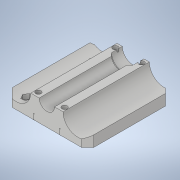
# Autodesk Inventor part: MINI-z-carriage-rear
Saved by Autodesk Inventor 2021 (Build 250183000, 183)
## iProperties
Company: Prusa Development a.s.
RuleStatus: InUse
Created: 2019-07-11
Material: Všeobecné
Document SubType Name: Modeling
Density: 1 g/cm^3
Appearance: Výchozí
Project: ORIGINAL PRUSA MINI
Authority: Ing. Robert Turinský
Author: Ing. Robert Turinský
Title: MINI-z-carriage-rear
Revision Number: R4
Autodesk Inventor part; units mm, degrees
ref_plane "YZ Plane" through (0, 0, 0) normal (1, 0, 0) x (0, 1, 0)
ref_plane "XZ Plane" through (0, 0, 0) normal (0, 1, 0) x (-1, 0, 0)
sketch "Náčrt1" plane through (0, 0, 0) normal (0, 0, 1) x (1, 0, 0)
  line L0 (0, -16.8) -> (0, 2.8) projected
  line L1 (-37.1, 0) -> (37.1, 0) projected
  arc A0 (-5, 0) -> (5, 0) centre (0, 0) ccw
  arc A1 (-26.5, -6.9282) -> (-10.5, 0) centre (-20, 0) ccw
  arc A2 (10.5, 0) -> (26.5, -6.9282) centre (20, 0) ccw
  line L2 (-10.5, 0) -> (-5, 0)
  line L3 (5, 0) -> (10.5, 0)
  line L4 (-26.5, -6.9282) -> (-26.5, -14)
  line L5 (-26.5, -14) -> (26.5, -14)
  line L6 (26.5, -14) -> (26.5, -6.9282)
  dimension "d0" = 19
  dimension "d1" = 10
  dimension "d2" = 40
  dimension "d3" = 53
  dimension "d4" = 14
  constraints: 10 end point, 6 point on circle, 3 centre point, 2 vertical, 1 coincident, 1 equal radius, 1 horizontal, 1 symmetric about line, 8 other
  measures "d0" diameter of A1
  measures "d1" diameter of A0
  measures "d2" distance of A2.centre A1.centre
  measures "d3" distance between parallel lines of L6 L4
  measures "d4" distance of the line from the sketch origin of L5
extrude "Vysunutí1" add sketch "Náčrt1" along normal mid plane 56 contours L5 L4 A1 L1 A0 L0 | L0 A0 L1 A2 L6 L5
sketch "Náčrt2" plane through (0, 0, -28) normal (0, 0, -1) x (-1, 0, 0)
  circle A0 centre (0, 0) radius 7
  point P0 (0, -9.5)
  dimension "d7" = 14
  dimension "d13" = 9.5
  constraints: 1 centre point, 1 coincident, 1 vertical alignment
  measures "d7" diameter of A0
  measures "d13" distance of point (0, 0) point (0, -9.5)
extrude "Vysunutí2" cut sketch "Náčrt2" against normal blind 7
chamfer "Zkosení1" distance 2 angle 45 1 edges at (0, -5, -21)
hole "Díra1" at (0, -9.5, -28) direction (0, 0, 1) diameter 3.4 depth 16 countersink diameter 4 countersink angle 60
sketch "Náčrt4" plane through (-26.5, -14, 28) normal (0, -1, 0) x (1, 0, 0)
  line L0 (26.5, -67.2) -> (26.5, 11.2) projected
  line L1 (-10.6, -28) -> (63.6, -28) projected
  line L2 (53, -56) -> (0, -56) projected
  line L3 (0, 0) -> (53, 0) projected
  point P0 (26.5, -28)
  point P1 (18, -3)
  point P2 (35, -3)
  point P3 (18, -53)
  point P4 (35, -53)
  dimension "d24" = 17
  dimension "d25" = 3
  dimension "d121" = 50
  constraints: 2 symmetric about line, 1 vertical alignment
  measures "d24" distance of point (35, -53) point (18, -53)
  measures "d25" distance from line of point (35, -53) L2
  measures "d121" distance of point (35, -3) point (35, -53)
hole "Díra2" at (-8.5, -14, 25) at (8.5, -14, 25) at (-8.5, -14, -25) at (8.5, -14, -25) direction (0, 1, 0) diameter 3.4 end through all counterbore diameter 6 counterbore depth 4.1
ref_plane "Pracovní rovina1" through (-26.5, -12.5, 28) normal (0, -1, 0) x (1, 0, 0)
sketch "Náčrt5" plane through (-26.5, -12.5, 28) normal (0, -1, 0) x (1, 0, 0)
  line L0 (26.5, -67.2) -> (26.5, 11.2) projected
  line L1 (-10.6, -28) -> (63.6, -28) projected
  circle A0 centre (8, -6) radius 1.7
  line L2 (0, 0) -> (53, 0) projected
  circle A1 centre (9.5, -48) radius 1.7
  line L3 (9.6166, -3.2) -> (11.2332, -6)
  line L4 (11.2332, -6) -> (9.6166, -8.8)
  line L5 (9.6166, -8.8) -> (6.3834, -8.8)
  line L6 (6.3834, -8.8) -> (4.7668, -6)
  line L7 (4.7668, -6) -> (6.3834, -3.2)
  line L8 (6.3834, -3.2) -> (9.6166, -3.2)
  line L9 (11.1166, -45.2) -> (12.7332, -48)
  line L10 (12.7332, -48) -> (11.1166, -50.8)
  line L11 (11.1166, -50.8) -> (7.8834, -50.8)
  line L12 (7.8834, -50.8) -> (6.2668, -48)
  line L13 (6.2668, -48) -> (7.8834, -45.2)
  line L14 (7.8834, -45.2) -> (11.1166, -45.2)
  point P0 (26.5, -28)
  dimension "d35" = 3.4
  dimension "d36" = 18.5
  dimension "d37" = 6
  dimension "d38" = 42
  dimension "d39" = 17
  dimension "d40" = 5.6
  constraints: 24 end point, 2 centre point, 2 coincident, 2 horizontal, 1 equal radius, 1 parallel, 26 other
  measures "d35" diameter of A0
  measures "d36" distance from line of L0 A0.centre
  measures "d37" distance from line of L2 A0.centre
  measures "d38" vertical distance of A1.centre A0.centre
  measures "d39" distance from line of L0 A1.centre
  measures "d40" distance between parallel lines of L5 L8
extrude "Vysunutí3" cut sketch "Náčrt5" along normal through all contours A0 | A1
extrude "Vysunutí4" cut sketch "Náčrt5" against normal through all contours A0 | A1 | L3 L4 L5 L6 L7 L8 | L9 L10 L11 L12 L13 L14
sketch "Náčrt6" plane through (-26.5, -14, 28) normal (0, -1, 0) x (1, 0, 0)
  circle A0 centre (47.5, -11) radius 3.25
  circle A1 centre (41.9, -44.9) radius 1.5
  circle A2 centre (4.5, -12) radius 1.5
  line L0 (26.5, -67.2) -> (26.5, 11.2) projected
  line L1 (-10.6, -28) -> (63.6, -28) projected
  line L2 (0, 0) -> (53, 0) projected
  point P0 (26.5, -28)
  dimension "d45" = 6.5
  dimension "d46" = 22
  dimension "d47" = 12
  dimension "d48" = 3
  dimension "d49" = 21
  dimension "d50" = 11
  dimension "d51" = 15.4
  dimension "d52" = 44.9
  dimension "d53" = 3
  constraints: 3 centre point
  measures "d45" diameter of A0
  measures "d46" distance from line of L0 A2.centre
  measures "d47" distance from line of A2.centre L2
  measures "d48" diameter of A2
  measures "d49" distance from line of L0 A0.centre
  measures "d50" distance from line of L2 A0.centre
  measures "d51" distance from line of L0 A1.centre
  measures "d52" distance from line of L2 A1.centre
  measures "d53" diameter of A1
extrude "Vysunutí5" cut sketch "Náčrt6" against normal blind 2 contours A1 | A2
extrude "Vysunutí6" cut sketch "Náčrt6" against normal blind 3 contours A0
chamfer "Zkosení2" distance 4 angle 45 2 edges at (-26.5, -10.4641, 28) (26.5, -10.4641, 28)
chamfer "Zkosení3" distance 5.5 angle 45 1 edges at (26.5, -10.4641, -28)
chamfer "Zkosení4" distance 1.5 angle 45 1 edges at (-26.5, -10.4641, -28)
ref_plane "Pracovní rovina2" through (0, 0, -18) normal (0, 0, -1) x (-1, 0, 0)
sketch "Náčrt7" plane through (0, 0, -18) normal (0, 0, -1) x (-1, 0, 0)
  line L0 (-17.75, -14) -> (-24.25, -14) projected
  line L1 (-13.9, -14) -> (-16.9, -14) projected
  line L2 (23.5, -14) -> (20.5, -14) projected
  line L3 (20.2, -14) -> (16.8, -14) projected
  line L4 (18.7, -14) -> (15.3, -14) projected
  line L5 (11.5, -14) -> (5.5, -14) projected
  line L6 (11.5, -14) -> (5.5, -14) projected
  line L7 (-5.5, -14) -> (-11.5, -14) projected
  line L8 (-5.5, -14) -> (-11.5, -14) projected
  line L9 (25, -14) -> (26.5, -14) projected
  line L10 (-21, -14) -> (-8.5, -14) projected
  line L11 (-26.5, -14) -> (-21, -14) projected
  line L12 (-22.5, -14) -> (-26.5, -14) projected
  line L13 (22.5, -14) -> (8.5, -14) projected
  line L14 (26.5, -14) -> (22.5, -14) projected
  circle A0 centre (0, -9.5) radius 1.7 projected
  line L15 (22.5, -14) -> (-22.5, -14) projected
  line L16 (2.8, -14) -> (-2.8, -14)
  line L17 (-2.8, -14) -> (-2.8, -6.7)
  line L18 (-2.8, -6.7) -> (2.8, -6.7)
  line L19 (2.8, -6.7) -> (2.8, -14)
  line L20 (2.8, -14) -> (1.7, -14)
  line L21 (1.7, -14) -> (1.7, -6.7)
  line L22 (1.7, -6.7) -> (2.8, -6.7)
  line L23 (2.8, -6.7) -> (2.8, -14)
  line L24 (2.8, -6.7) -> (-2.8, -6.7)
  line L25 (-2.8, -6.7) -> (-2.8, -7.8)
  line L26 (-2.8, -7.8) -> (2.8, -7.8)
  line L27 (2.8, -7.8) -> (2.8, -6.7)
  line L28 (-2.8, -6.7) -> (-1.7, -6.7)
  line L29 (-1.7, -6.7) -> (-1.7, -14)
  line L30 (-1.7, -14) -> (-2.8, -14)
  line L31 (-2.8, -14) -> (-2.8, -6.7)
  line L32 (-2.8, -14) -> (2.8, -14)
  line L33 (2.8, -14) -> (2.8, -11.2)
  line L34 (2.8, -11.2) -> (-2.8, -11.2)
  line L35 (-2.8, -11.2) -> (-2.8, -14)
  line L36 (-8.5, -14) -> (-22.5, -14) projected
  line L37 (8.5, -14) -> (-8.5, -14) projected
  line L38 (8.5, -14) -> (25, -14) projected
  line L39 (-8.5, -14) -> (8.5, -14) projected
  point P0 (0, 0)
  point P1 (0, -14)
  dimension "d68" = 5.6
  dimension "d69" = 2.8
  constraints: 40 end point, 10 parallel, 5 horizontal, 5 perpendicular, 4 point on line, 4 tangent, 1 midpoint, 1 vertical alignment, 2 other
  measures "d68" distance of L17.end L18.end
  measures "d69" distance from line of L18 A0.centre
extrude "Vysunutí7" cut sketch "Náčrt7" along normal blind 2.6
extrude "Vysunutí8" add sketch "Náčrt7" along normal blind 0.3 contours L21 L26 L19 L34 | L34 L19 L15 L21 | L21 L18 L19 L26 | L29 L34 L17 L26 | L26 L17 L18 L29 | L29 L15 L17 L34
extrude "Vysunutí9" add sketch "Náčrt7" along normal blind 0.6 contours L26 L29 L18 L21 | L34 L21 L15 L29 | L34 L19 L15 L21 | L21 L18 L19 L26 | L26 L17 L18 L29 | L29 L15 L17 L34
chamfer "Zkosení5" distance 0.5 angle 60 4 edges at (2.8, -14, -19.6) (0, -14, -20.6) (-2.8, -14, -19.6) (0, -14, -18.6) measured on face at (0, -14, -18.5) measured on face at (0, -14, -21.1) measured on face at (-3.3, -14, -19.6) measured on face at (3.3, -14, -19.6)
ref_plane "Pracovní rovina3" through (0, 0, 16) normal (0, 0, 1) x (1, 0, 0)
sketch "Náčrt8" plane through (0, 0, 16) normal (0, 0, 1) x (1, 0, 0)
  line L0 (24.25, -14) -> (17.75, -14) projected
  line L1 (16.9, -14) -> (13.9, -14) projected
  line L2 (-20.5, -14) -> (-23.5, -14) projected
  line L3 (-16.8, -14) -> (-20.2, -14) projected
  line L4 (-15.3, -14) -> (-18.7, -14) projected
  line L5 (-5.5, -14) -> (-11.5, -14) projected
  line L6 (-5.5, -14) -> (-11.5, -14) projected
  line L7 (11.5, -14) -> (5.5, -14) projected
  line L8 (11.5, -14) -> (5.5, -14) projected
  line L9 (-25, -14) -> (-26.5, -14) projected
  line L10 (21, -14) -> (8.5, -14) projected
  line L11 (26.5, -14) -> (21, -14) projected
  line L12 (22.5, -14) -> (26.5, -14) projected
  line L13 (-22.5, -14) -> (-8.5, -14) projected
  line L14 (-26.5, -14) -> (-22.5, -14) projected
  line L15 (-3.3, -14) -> (3.3, -14) projected
  line L16 (3.3, -14) -> (-3.3, -14) projected
  line L17 (0, -16.8003) -> (0, 2.8017) projected
  line L18 (-37.1, 0) -> (37.1, 0) projected
  line L19 (-2, -12) -> (-2, -14)
  line L20 (-2, -14) -> (-9.75, -14)
  line L21 (21, -14) -> (-25, -14) projected
  line L22 (-9.75, -14) -> (-8.5953, -12)
  line L23 (-8.5953, -12) -> (-2, -12)
  line L24 (8.5, -14) -> (22.5, -14) projected
  line L25 (-8.5, -14) -> (8.5, -14) projected
  line L26 (-8.5, -14) -> (-25, -14) projected
  line L27 (8.5, -14) -> (-8.5, -14) projected
  line L28 (-9.75, -14) -> (-10.9047, -14)
  line L29 (-10.9047, -14) -> (-9.1726, -11)
  line L30 (-9.1726, -11) -> (-2, -11)
  line L31 (-2, -11) -> (-2, -12)
  point P0 (0, 0)
  dimension "d80" = 2
  dimension "d85" = 2
  dimension "d127" = 15.5
  dimension "d128" = 60
  dimension "d139" = 1
  dimension "d140" = 1
  constraints: 16 end point, 3 point on line, 2 parallel, 2 perpendicular, 1 horizontal, 1 other
  measures "d80" distance between parallel lines of L17 L19
  measures "d85" distance between parallel lines of L13 L23
  measures "d127" diameter of L20.end L19
  measures "d128" angle of L5 L22
  measures "d139" distance between parallel lines of L30 L23
  measures "d140" distance between parallel lines of L29 L22
revolve "Rotace1" cut sketch "Náčrt8" angle 360 about axis through (-2, -12, 16) along (0, -1, 0) contours L5 L22 L23 L19 L15 L20
sketch "Náčrt9" plane through (-22.5, -14, 28) normal (0, -1, 0) x (1, 0, 0)
  line L0 (22.5, -67.2) -> (22.5, 11.2) projected
  line L1 (-14.6, -28) -> (59.6, -28) projected
  line L2 (10.878, -17.017) -> (34.122, -17.017) construction
  line L3 (34.122, -17.017) -> (34.122, -38.983) construction
  line L4 (34.122, -38.983) -> (10.878, -38.983) construction
  line L5 (10.878, -38.983) -> (10.878, -17.017) construction
  point P0 (22.5, -28)
  constraints: 4 other
feature "Reliéf1" [suppressed]
chamfer "Zkosení6" [suppressed]
chamfer "Zkosení7" [suppressed]
feature "Reliéf2" [suppressed]
sketch "Náčrt11" plane through (8.5, -9.9, -25) normal (0, -1, 0) x (1, 0, 0)
  circle A0 centre (0, 0) radius 3 projected
  circle A1 centre (0, 0) radius 1.7 projected
  circle A2 centre (-17, 0) radius 3 projected
  circle A3 centre (-17, 0) radius 1.7 projected
  circle A4 centre (-17, 50) radius 3 projected
  circle A5 centre (-17, 50) radius 1.7 projected
  circle A6 centre (0, 50) radius 3 projected
  circle A7 centre (0, 50) radius 1.7 projected
  line L0 (1.7, -2.4718) -> (1.7, 2.4718)
  line L1 (-1.7, 2.4718) -> (-1.7, -2.4718)
  line L2 (-2.4718, -1.7) -> (2.4718, -1.7)
  line L3 (2.4718, 1.7) -> (-2.4718, 1.7)
  arc A8 (1.7, -2.4718) -> (1.7, 2.4718) centre (0, 0) ccw
  arc A9 (2.4718, 1.7) -> (-2.4718, 1.7) centre (0, 0) ccw
  arc A10 (-1.7, 2.4718) -> (-1.7, -2.4718) centre (0, 0) ccw
  arc A11 (-2.4718, -1.7) -> (2.4718, -1.7) centre (0, 0) ccw
  point P0 (-8.5, 25)
  point P1 (0, 53)
  point P2 (-17, 53)
  point P3 (-17, -3)
  point P4 (0, -3)
  constraints: 12 point on circle, 8 end point, 4 centre point, 4 tangent, 3 vertical alignment, 2 perpendicular, 2 vertical, 9 other
extrude "Vysunutí10" add sketch "Náčrt11" along normal blind 0.3 contours A0 L2 L0 L3 | L3 L0 A0 | A0 L0 L2 | L1 L3 A0 | A0 L2 L1 | L3 L1 L2 A0
extrude "Vysunutí11" add sketch "Náčrt11" along normal blind 0.6 contours L3 L0 A0 | A0 L0 L2 | L0 L3 L1 A0 | A0 L1 L2 L0 | L1 L3 A0 | A0 L2 L1
pattern_linear "Obdélníkové pole1" count 2 spacing 17 along (-1, 0, 0) count 2 spacing 50 along (0, 0, 1) of "Vysunutí11", "Vysunutí10"
sketch "Náčrt10" plane through (0, 0, -28) normal (0, 0, -1) x (-1, 0, 0)
  line L0 (25, -8.0777) -> (25, -14) projected
  arc A0 (10.5, 0) -> (25, -8.0777) centre (20, 0) ccw projected
  circle A1 centre (0, -9.5) radius 2 projected
  arc A2 (-21, -9.4472) -> (-10.5, 0) centre (-20, 0) ccw projected
  line L1 (-21, -14) -> (-21, -9.4472) projected
  line L2 (-10.5, -7.25) -> (-5.5, -7.25) construction
  line L3 (-5.5, -7.25) -> (-5.5, -12.25) construction
  line L4 (-5.5, -12.25) -> (-10.5, -12.25) construction
  line L5 (-10.5, -12.25) -> (-10.5, -7.25) construction
  line L6 (10.5, 0) -> (7, 0) projected
  arc A3 (-7, 0) -> (7, 0) centre (0, 0) ccw projected
  line L7 (-7, 0) -> (-10.5, 0) projected
  line L8 (-21, -14) -> (-8.5, -14) projected
  line L9 (-8.5, -9.9) -> (-8.5, -14) projected
  line L10 (-8.5, -14) -> (8.5, -14) projected
  line L11 (8.5, -9.9) -> (8.5, -14) projected
  line L12 (8.5, -14) -> (25, -14) projected
  dimension "d95" = 5
  dimension "d97" = 5.5
  constraints: 1 perpendicular, 2 other
  measures "d95" distance of L3.end L4.end
  measures "d97" distance from line of point (0, 0) L3
move faces "Posunout2" translate (0, -2, 0) faces at (-21.8227, -12, 15.5325) (15.8427, -12, -17.1324)
move faces "Posunout3" translate (-1, 0, 0) faces at (24.2395, -13, 17.2615) (19.4208, -11, 16.2816)
sketch "Náčrt12" plane through (-8.5, -14, -28) normal (0, -1, 0) x (1, 0, 0)
  line L0 (8.5, -11.2) -> (8.5, 67.2) projected
  line L1 (-28.6, 28) -> (45.6, 28) projected
  line L2 (-1.9595, 37.5892) -> (18.9595, 37.5892) construction
  line L3 (18.9595, 37.5892) -> (18.9595, 18.4108) construction
  line L4 (18.9595, 18.4108) -> (-1.9595, 18.4108) construction
  line L5 (-1.9595, 18.4108) -> (-1.9595, 37.5892) construction
  line L6 (9.0412, 25.0123) -> (7.2112, 25.0123)
  line L7 (7.2112, 25.0123) -> (5.5463, 27.2112)
  line L8 (5.5463, 27.2112) -> (5.0026, 27.2112)
  line L9 (5.0026, 27.2112) -> (5.0026, 25.0123)
  line L10 (5.0026, 25.0123) -> (3.5075, 25.0123)
  line L11 (3.5075, 25.0123) -> (3.5075, 31.0023)
  line L12 (3.5075, 31.0023) -> (5.9152, 31.0023)
  spline S0 degree 2 poles (5.9152, 31.0023) (6.4152, 31.0023) (7.153, 30.8761) (7.4685, 30.6819) knots 0 0 0 1 2 2 2
  spline S1 degree 2 poles (7.4685, 30.6819) (7.7889, 30.478) (8.1675, 29.8421) (8.1675, 29.3567) knots 0 0 0 1 2 2 2
  spline S2 degree 2 poles (8.1675, 29.3567) (8.1675, 28.6723) (7.5462, 27.8131) (7.0268, 27.5607) knots 0 0 0 1 2 2 2
  line L13 (7.0268, 27.5607) -> (9.0412, 25.0123)
  spline S3 degree 2 poles (6.6239, 29.1674) (6.6239, 29.3956) (6.4491, 29.7208) (6.2501, 29.8082) knots 0 0 0 1 2 2 2
  spline S4 degree 2 poles (6.2501, 29.8082) (6.1093, 29.8664) (5.7647, 29.9004) (5.5074, 29.9004) knots 0 0 0 1 2 2 2
  line L14 (5.5074, 29.9004) -> (5.0026, 29.9004)
  line L15 (5.0026, 29.9004) -> (5.0026, 28.2888)
  line L16 (5.0026, 28.2888) -> (5.4346, 28.2888)
  spline S5 degree 2 poles (5.4346, 28.2888) (5.7453, 28.2888) (6.187, 28.3665) (6.3375, 28.4878) knots 0 0 0 1 2 2 2
  spline S6 degree 2 poles (6.3375, 28.4878) (6.4831, 28.6043) (6.6239, 28.915) (6.6239, 29.1674) knots 0 0 0 1 2 2 2
  line L17 (13.9488, 26.4103) -> (13.1381, 26.4103)
  line L18 (13.1381, 26.4103) -> (13.1381, 24.9977)
  line L19 (13.1381, 24.9977) -> (11.6867, 24.9977)
  line L20 (11.6867, 24.9977) -> (11.6867, 26.4103)
  line L21 (11.6867, 26.4103) -> (9.0461, 26.4103)
  line L22 (9.0461, 26.4103) -> (9.0461, 27.5267)
  line L23 (9.0461, 27.5267) -> (11.6382, 31.0023)
  line L24 (11.6382, 31.0023) -> (13.1381, 31.0023)
  line L25 (13.1381, 31.0023) -> (13.1381, 27.4879)
  line L26 (13.1381, 27.4879) -> (13.9488, 27.4879)
  line L27 (13.9488, 27.4879) -> (13.9488, 26.4103)
  line L28 (11.6867, 27.4879) -> (11.6867, 29.5266)
  line L29 (11.6867, 29.5266) -> (10.1674, 27.4879)
  line L30 (10.1674, 27.4879) -> (11.6867, 27.4879)
  point P0 (8.5, 28)
  dimension "rev_num" = 4
  constraints: 4 other
emboss "Reliéf3" sketch "Náčrt12" operation cut depth 0.75 direction (0, 1, 0) contours L6 L7 L8 L9 L10 L11 L1 S2 L13 L0 | L0 L13 L6 | L1 L11 L12 S0 S1 S2 | L23 L24 L25 L1 L28 L29 | L1 L29 L30 L28 L25 L26 L27 L17 L18 L19 L20 L21 L22 L23
move faces "Posunout4" translate (0, 0, 6.1) faces at (0, -12.4893, -20.6) (-0.9333, -13.7113, -20.9333) (3.1333, -13.7113, -19.9333) (2.8, -10.3447, -19.9333) (-0.9333, -13.7113, -18.2667) (-3.1333, -13.7113, -19.9333) (-0.9333, -6.7, -19.9333) (-2.8, -10.3447, -19.9333) (-0.9333, -7.4333, -18.6) (-0.5667, -7.8, -18.5) (-2.0667, -8.9333, -18.3) (0.9333, -12.4893, -18.6) (-1.7, -9.5, -18.2) (0.5667, -11.2, -18.5) (2.0667, -10.0667, -18.3) (1.7, -9.5, -18.2) (1.363, -10.863, -18) (1.363, -8.137, -18) (-1.363, -8.137, -18) (-1.363, -10.863, -18)
chamfer "Zkosení8" distance 1 angle 45 1 edges at (16.75, -11, 17)
ref_plane "Pracovní rovina4" through (0, 0, -10) normal (0, 0, 1) x (1, 0, 0)
sketch "Náčrt13" plane through (0, 0, -10) normal (0, 0, 1) x (1, 0, 0)
  line L0 (22.5, -9.1652) -> (22.5, -14) projected
  arc A0 (10.5, 0) -> (22.5, -9.1652) centre (20, 0) ccw projected
  line L1 (10.5, 0) -> (5, 0) projected
  arc A1 (-5, 0) -> (5, 0) centre (0, 0) ccw projected
  line L2 (-5, 0) -> (-10.5, 0) projected
  arc A2 (-22.5, -9.1652) -> (-10.5, 0) centre (-20, 0) ccw projected
  line L3 (-22.5, -14) -> (-22.5, -9.1652) projected
  line L4 (-22.5, -14) -> (-8.5, -14) projected
  line L5 (-8.5, -10.5) -> (-8.5, -14) projected
  line L6 (-8.5, -14) -> (8.5, -14) projected
  line L7 (8.5, -10.5) -> (8.5, -14) projected
  line L8 (8.5, -14) -> (22.5, -14) projected
  arc A3 (22.5, -9.1652) -> (26.5, -6.9282) centre (20, 0) ccw projected
  line L9 (22.5, -9.1652) -> (22.5, -14) projected
  line L10 (22.5, -14) -> (26.5, -14) projected
  line L11 (26.5, -14) -> (26.5, -6.9282) projected
  line L12 (-26.5, -14) -> (-22.5, -14) projected
  line L13 (-22.5, -14) -> (-22.5, -9.1652) projected
  arc A4 (-26.5, -6.9282) -> (-22.5, -9.1652) centre (-20, 0) ccw projected
  line L14 (-26.5, -6.9282) -> (-26.5, -14) projected
  line L15 (8.5, -13) -> (21.5, -13)
  line L16 (21.5, -13) -> (21.5, -10.3923)
  arc A5 (9.5477, -1) -> (21.5, -10.3923) centre (20, 0) ccw
  line L17 (9.5477, -1) -> (5.9161, -1)
  arc A6 (-5.9161, -1) -> (5.9161, -1) centre (0, 0) ccw
  line L18 (-5.9161, -1) -> (-9.5477, -1)
  arc A7 (-21.5, -10.3923) -> (-9.5477, -1) centre (-20, 0) ccw
  line L19 (-21.5, -10.3923) -> (-21.5, -13)
  line L20 (-21.5, -13) -> (-8.5, -13)
  line L21 (8.5, -13) -> (-8.5, -13)
  line L22 (-23.5, -9.8995) -> (-23.5, -13)
  line L23 (-23.5, -13) -> (-25.5, -13)
  line L24 (-25.5, -13) -> (-25.5, -8.9443)
  arc A8 (-25.5, -8.9443) -> (-23.5, -9.8995) centre (-20, 0) ccw
  arc A9 (23.5, -9.8995) -> (25.5, -8.9443) centre (20, 0) ccw
  line L25 (23.5, -9.8995) -> (23.5, -13)
  line L26 (23.5, -13) -> (25.5, -13)
  line L27 (25.5, -13) -> (25.5, -8.9443)
  arc A10 (21.5, -10.3923) -> (23.5, -9.8995) centre (20, 0) ccw
  arc A11 (-23.5, -9.8995) -> (-21.5, -10.3923) centre (-20, 0) ccw
  line L28 (-21.5, -13) -> (-23.5, -13)
  line L29 (23.5, -13) -> (21.5, -13)
  dimension "d133" = 1
  constraints: 30 end point, 14 point on circle, 7 centre point, 4 concentric, 2 collinear, 1 horizontal, 14 other
  measures "d133" distance between parallel lines of L8 L15
extrude "Vysunutí12" cut sketch "Náčrt13" along normal mid plane 0.1 contours A10 L25 L29 L0 | L0 L29 L16 A10 | L16 L15 L21 L20 L19 A7 L18 A6 L17 A5 | A9 L27 L26 L25 | L28 L3 A11 L19 | L3 L28 L22 A11 | L22 L23 L24 A8
pattern_linear "Obdélníkové pole2" count 5 spacing 5 along (0, 0, 1) of "Vysunutí12"
revolve "Rotace2" add sketch "Náčrt8" angle 360 about axis through (-2, -12, 16) along (0, -1, 0) contours L5 L29 L30 L31 L23 L22
sketch "Náčrt15" plane through (0, 0, 0) normal (0, 0, 1) x (1, 0, 0)
  arc A0 (-25, -8.0777) -> (-10.5, 0) centre (-20, 0) ccw projected
  arc A1 (-25.5263, -8.928) -> (-9.5, 0) centre (-20, 0) ccw
  point P0 (0, 0)
  dimension "d144" = 1
  constraints: 2 point on circle, 1 centre point
  measures "d144" radial gap between concentric circles of A0 A1
surface extrude "VysunutíDoPlochy1" sketch "Náčrt15" along normal mid plane 56 shown no curves A1
sketch "Náčrt14" plane through (-26.5, -12.5, 28) normal (0, 1, 0) x (1, 0, 0)
  circle A0 centre (8, 6) radius 1.7 projected
  line L0 (9.6166, 3.2) -> (11.2332, 6) projected
  line L1 (11.2332, 6) -> (9.6166, 8.8) projected
  line L2 (9.6166, 8.8) -> (6.3834, 8.8) projected
  line L3 (6.3834, 8.8) -> (4.7668, 6) projected
  line L4 (4.7668, 6) -> (6.3834, 3.2) projected
  line L5 (6.3834, 3.2) -> (9.6166, 3.2) projected
  circle A1 centre (9.5, 48) radius 1.7 projected
  line L6 (11.1166, 45.2) -> (12.7332, 48) projected
  line L7 (12.7332, 48) -> (11.1166, 50.8) projected
  line L8 (11.1166, 50.8) -> (7.8834, 50.8) projected
  line L9 (7.8834, 50.8) -> (6.2668, 48) projected
  line L10 (6.2668, 48) -> (7.8834, 45.2) projected
  line L11 (7.8834, 45.2) -> (11.1166, 45.2) projected
  line L12 (5.8927, 2.35) -> (3.7853, 6)
  line L13 (3.7853, 6) -> (5.8927, 9.65)
  line L14 (5.8927, 9.65) -> (10.1073, 9.65)
  line L15 (10.1073, 9.65) -> (12.2147, 6)
  line L16 (12.2147, 6) -> (10.1073, 2.35)
  line L17 (10.1073, 2.35) -> (5.8927, 2.35)
  line L18 (7.3927, 44.35) -> (5.2853, 48)
  line L19 (5.2853, 48) -> (7.3927, 51.65)
  line L20 (7.3927, 51.65) -> (11.6073, 51.65)
  line L21 (11.6073, 51.65) -> (13.7147, 48)
  line L22 (13.7147, 48) -> (11.6073, 44.35)
  line L23 (11.6073, 44.35) -> (7.3927, 44.35)
  line L24 (3.6699, 6) -> (5.8349, 2.25)
  line L25 (5.8349, 2.25) -> (10.1651, 2.25)
  line L26 (10.1651, 2.25) -> (12.3301, 6)
  line L27 (12.3301, 6) -> (10.1651, 9.75)
  line L28 (10.1651, 9.75) -> (5.8349, 9.75)
  line L29 (5.8349, 9.75) -> (3.6699, 6)
  line L30 (5.1699, 48) -> (7.3349, 44.25)
  line L31 (7.3349, 44.25) -> (11.6651, 44.25)
  line L32 (11.6651, 44.25) -> (13.8301, 48)
  line L33 (13.8301, 48) -> (11.6651, 51.75)
  line L34 (11.6651, 51.75) -> (7.3349, 51.75)
  line L35 (7.3349, 51.75) -> (5.1699, 48)
  line L36 (5.3442, 1.4) -> (2.6884, 6)
  line L37 (2.6884, 6) -> (5.3442, 10.6)
  line L38 (5.3442, 10.6) -> (10.6558, 10.6)
  line L39 (10.6558, 10.6) -> (13.3116, 6)
  line L40 (13.3116, 6) -> (10.6558, 1.4)
  line L41 (10.6558, 1.4) -> (5.3442, 1.4)
  line L42 (2.5729, 6) -> (5.2865, 1.3)
  line L43 (5.2865, 1.3) -> (10.7135, 1.3)
  line L44 (10.7135, 1.3) -> (13.4271, 6)
  line L45 (13.4271, 6) -> (10.7135, 10.7)
  line L46 (10.7135, 10.7) -> (5.2865, 10.7)
  line L47 (5.2865, 10.7) -> (2.5729, 6)
  line L48 (6.8442, 43.4) -> (4.1884, 48)
  line L49 (4.1884, 48) -> (6.8442, 52.6)
  line L50 (6.8442, 52.6) -> (12.1558, 52.6)
  line L51 (12.1558, 52.6) -> (14.8116, 48)
  line L52 (14.8116, 48) -> (12.1558, 43.4)
  line L53 (12.1558, 43.4) -> (6.8442, 43.4)
  line L54 (4.0729, 48) -> (6.7865, 43.3)
  line L55 (6.7865, 43.3) -> (12.2135, 43.3)
  line L56 (12.2135, 43.3) -> (14.9271, 48)
  line L57 (14.9271, 48) -> (12.2135, 52.7)
  line L58 (12.2135, 52.7) -> (6.7865, 52.7)
  line L59 (6.7865, 52.7) -> (4.0729, 48)
  point P0 (26.5, 28)
  dimension "d142" = 0.85
  dimension "d143" = 0.1
  dimension "d149" = 0.1
  dimension "d150" = 0.85
  constraints: 96 end point, 4 parallel, 40 other
  measures "d142" distance between parallel lines of L4 L12
  measures "d143" distance between parallel lines of L12 L24
  measures "d149" distance between parallel lines of L42 L36
  measures "d150" distance between parallel lines of L36 L24
extrude "Vysunutí13" add sketch "Náčrt14" along normal up to surface separate body contours L12 L13 L14 L15 L16 L17 | L18 L19 L20 L21 L22 L23 | L29 L28 L27 L26 L25 L24 | L35 L34 L33 L32 L31 L30 | L36 L37 L38 L39 L40 L41 | L47 L46 L45 L44 L43 L42 | L48 L49 L50 L51 L52 L53 | L59 L58 L57 L56 L55 L54 round surface about axis through (-20, 0, 0) along (0, 0, 1) radius 10.5 far side no
sketch "Náčrt16" plane through (-8.5, -14, -28) normal (0, -1, 0) x (1, 0, 0)
  circle A0 centre (6.5, 44) radius 7.75 projected
  arc A1 (0, 56) -> (-0.0788, 50.001) centre (0, 53) ccw projected
  line L0 (-14, 56) -> (0, 56) projected
  line L1 (-18, 52) -> (-14, 56) projected
  line L2 (-18, 1.5) -> (-18, 52) projected
  line L3 (-16.5, 0) -> (-18, 1.5) projected
  line L4 (0, 0) -> (-16.5, 0) projected
  circle A2 centre (0, 3) radius 3 projected
  line L5 (17, 0) -> (0, 0) projected
  circle A3 centre (17, 3) radius 3 projected
  line L6 (29.5, 0) -> (17, 0) projected
  line L7 (35, 5.5) -> (29.5, 0) projected
  line L8 (35, 5.5) -> (35, 52) projected
  line L9 (31, 56) -> (35, 52) projected
  line L10 (17, 56) -> (31, 56) projected
  circle A4 centre (17, 53) radius 3 projected
  line L11 (0, 56) -> (17, 56) projected
  arc A5 (2.8717, 52.132) -> (0, 56) centre (0, 53) ccw projected
  arc A6 (2.8717, 52.132) -> (-0.0788, 50.001) centre (6.5, 44) ccw projected
  line L12 (8.1675, 29.8501) -> (7.0268, 29.8501) projected
  line L13 (8.1135, 30.6819) -> (8.1135, 29.3567) projected
  line L14 (5.9152, 30.9927) -> (7.4685, 30.9927) projected
  line L15 (3.5075, 31.0023) -> (5.9152, 31.0023) projected
  line L16 (5.0026, 25.0123) -> (3.5075, 25.0123) projected
  line L17 (5.0026, 27.2112) -> (5.0026, 25.0123) projected
  line L18 (5.5463, 27.2112) -> (5.0026, 27.2112) projected
  line L19 (7.2112, 25.0123) -> (5.5463, 27.2112) projected
  line L20 (9.0412, 25.0123) -> (7.2112, 25.0123) projected
  line L21 (7.0268, 27.5607) -> (9.0412, 25.0123) projected
  line L22 (6.3375, 31.0073) -> (6.6239, 31.0073) projected
  line L23 (11.7844, 29.1674) -> (11.7844, 29.8082) projected
  line L24 (6.2501, 26.0381) -> (5.5074, 26.0381) projected
  line L25 (5.5074, 29.9004) -> (5.0026, 29.9004) projected
  line L26 (5.0026, 29.9004) -> (5.0026, 28.2888) projected
  line L27 (5.0026, 28.2888) -> (5.4346, 28.2888) projected
  line L28 (13.5008, 28.2888) -> (13.5008, 28.4878) projected
  circle A7 centre (28.5, 45) radius 3.25 projected
  circle A8 centre (-10, 50) radius 1.7 projected
  circle A9 centre (-8.5, 8) radius 1.7 projected
  line L29 (11.8, 13) -> (11.8, 16) projected
  line L30 (5.2, 13) -> (11.8, 13) projected
  line L31 (5.2, 16) -> (5.2, 13) projected
  line L32 (11.8, 16) -> (5.2, 16) projected
  circle A10 centre (0, 53) radius 3
  line L33 (3.5075, 25.0123) -> (3.5075, 31.0023) projected
  point P0 (8.5, 28)
  point P1 (6.3375, 28.4878)
  point P2 (6.6239, 29.1674)
  point P3 (6.2501, 29.8082)
  point P4 (8.1675, 29.3567)
  point P5 (7.4685, 30.6819)
  constraints: 3 vertical alignment, 1 centre point, 1 coincident, 1 concentric, 7 other
extrude "Vysunutí14" cut sketch "Náčrt16" against normal up to surface (3.5 mm away) contours A5 A6 A1 | A6 A10
sketch "Náčrt17" plane through (0, -9.5, -12) normal (0, 0, -1) x (-0.7071068, 0.7071068, 0)
  arc A0 (1.2021, -1.2021) -> (1.2021, 1.2021) centre (0, 0) ccw projected
  arc A1 (1.2021, 1.2021) -> (-1.2021, 1.2021) centre (0, 0) ccw projected
  arc A2 (-1.2021, 1.2021) -> (-1.2021, -1.2021) centre (0, 0) ccw projected
  arc A3 (-1.2021, -1.2021) -> (1.2021, -1.2021) centre (0, 0) ccw projected
  point P0 (6.7175, 6.7175)
extrude "Vysunutí15" cut sketch "Náčrt17" against normal blind 2
equation "\"d10\" = -0.5 * d1 + 0.5 * d7"
equation "\"d139\" = d133"
equation "\"d140\" = d133"
equation "\"d106\" = d24"
equation "\"d109\" = d121"
equation "\"rev_num\" = 4"
equation "\"d144\" = d133"
equation "\"d145\" = d5"
equation "\"d149\" = d143"
equation "\"d150\" = d142"
equation "\"d5\" = 56"
